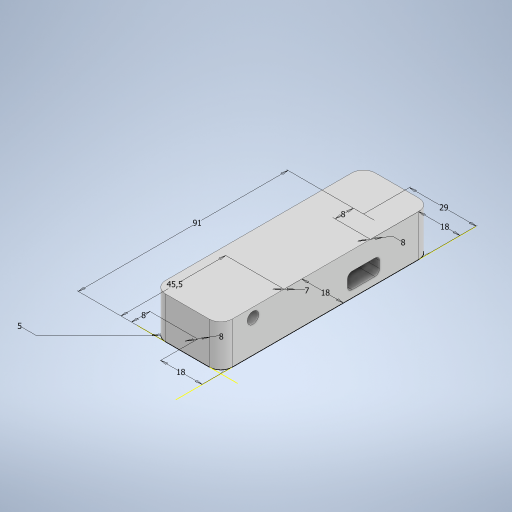
# Autodesk Inventor part: camera_model
Saved by Autodesk Inventor 2024.3 (Build 283343000, 343)
## iProperties
Created: 2026-05-02
Part Number: camera_model
Material: Generic
Document SubType Name: Modeling
Designer: owozn
Density: 1 g/cm^3
Appearance: Default
Author: owozn
Autodesk Inventor part; units mm, degrees
ref_plane "YZ Plane" through (0, 0, 0) normal (1, 0, 0) x (0, 1, 0)
ref_plane "XZ Plane" through (0, 0, 0) normal (0, 1, 0) x (-1, 0, 0)
ref_plane "XY Plane" through (0, 0, 0) normal (0, 0, 1) x (1, 0, 0)
sketch "Sketch1" plane through (0, 0, 0) normal (0, 1, 0) x (-1, 0, 0)
  line L0 (0, -110.6497) -> (0, 19.6497) projected
  line L1 (36.2497, 0) -> (-7.2497, 0) projected
  line L2 (5, 0) -> (24, 0)
  line L3 (29, -5) -> (29, -86)
  line L4 (24, -91) -> (5, -91)
  line L5 (0, -86) -> (0, -5)
  line L6 (0, 0) -> (29, -91) construction
  line L7 (29, 0) -> (0, -91) construction
  arc A0 (29, -5) -> (24, 0) centre (24, -5) ccw
  arc A1 (24, -91) -> (29, -86) centre (24, -86) ccw
  arc A2 (0, -86) -> (5, -91) centre (5, -86) ccw
  arc A3 (5, 0) -> (0, -5) centre (5, -5) ccw
  circle A4 centre (18, -8) radius 4
  circle A5 centre (18, -45.5) radius 3.5
  circle A6 centre (18, -83) radius 4
  point P0 (0, -5)
  dimension "d0" = 29
  dimension "d1" = 91
  dimension "d2" = 5
  dimension "d3" = 8
  dimension "d4" = 7
  dimension "d5" = 8
  dimension "d6" = 18
  dimension "d7" = 45.5
  dimension "d8" = 18
  dimension "d9" = 8
  dimension "d10" = 8
  dimension "d11" = 18
  constraints: 12 end point, 8 point on circle, 8 point on line, 8 tangent, 7 centre point, 3 equal radius, 2 parallel, 1 horizontal, 1 perpendicular
  measures "d0" distance of L6.end L7.end
  measures "d1" distance of L7.start L6.end
  measures "d2" radius of A0
  measures "d3" diameter of A4
  measures "d4" diameter of A5
  measures "d5" distance from line of L2 A4.centre
  measures "d6" distance from line of L5 A4.centre
  measures "d7" distance from line of L2 A5.centre
  measures "d8" distance from line of L5 A5.centre
  measures "d9" diameter of A6
  measures "d10" distance from line of L4 A6.centre
  measures "d11" distance from line of L5 A6.centre
extrude "Extrusion1" add sketch "Sketch1" along normal blind 18 contours L0 A3 L1 A0 L3 A1 L4 A2 | A4 | A5 | A6
sketch "Sketch2" plane through (0, 0, -5) normal (1, 0, 0) x (0, 0, -1)
  line L0 (-5, -3.6) -> (-5, 21.6) projected
  line L1 (104.2, 0) -> (-23.2, 0) projected
  circle A0 centre (9, 14) radius 2.5
  line L2 (52, 10) -> (62, 10)
  line L3 (64, 8) -> (64, 5)
  line L4 (62, 3) -> (52, 3)
  line L5 (50, 5) -> (50, 8)
  line L6 (50, 10) -> (64, 3) construction
  line L7 (64, 10) -> (50, 3) construction
  arc A1 (64, 8) -> (62, 10) centre (62, 8) ccw
  arc A2 (62, 3) -> (64, 5) centre (62, 5) ccw
  arc A3 (50, 5) -> (52, 3) centre (52, 5) ccw
  arc A4 (52, 10) -> (50, 8) centre (52, 8) ccw
  point P0 (-5, 0)
  point P1 (57, 6.5)
  point P2 (50, 6.5)
  dimension "d14" = 5
  dimension "d15" = 14
  dimension "d16" = 14
  dimension "d17" = 14
  dimension "d18" = 7
  dimension "d19" = 2
  dimension "d20" = 55
  dimension "d21" = 3
  constraints: 12 end point, 8 point on circle, 8 point on line, 8 tangent, 5 centre point, 3 equal radius, 3 midpoint, 2 parallel, 1 horizontal, 1 perpendicular
  measures "d14" diameter of A0
  measures "d15" distance from line of L0 A0.centre
  measures "d16" distance from line of L1 A0.centre
  measures "d17" distance of L6.end L7.end
  measures "d18" distance of L7.start L6.end
  measures "d19" radius of A1
  measures "d20" distance from line of L0 point (50, 6.5)
  measures "d21" distance between parallel lines of L1 L4
extrude "Extrusion2" cut sketch "Sketch1" along normal blind 2 contours A4 | A5 | A6
extrude "Extrusion3" cut sketch "Sketch2" against normal blind 8
body "Solid1"
